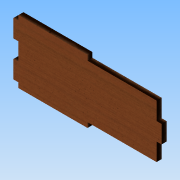
# Autodesk Inventor part: bottom2
Saved by Autodesk Inventor 2015 (Build 190159000, 159)
## iProperties
Created: 2015-12-28
Part Number: bottom2
Material: Générique
Document SubType Name: Modeling
Designer: Gregwar
Density: 1 g/cm^3
Appearance: Par défaut
Author: Gregwar
Autodesk Inventor part; units mm, degrees
ref_plane "YZ Plane" through (0, 0, 0) normal (1, 0, 0) x (0, 1, 0)
ref_plane "XZ Plane" through (0, 0, 0) normal (0, 1, 0) x (-1, 0, 0)
ref_plane "XY Plane" through (0, 0, 0) normal (0, 0, 1) x (1, 0, 0)
sketch "Esquisse1" plane through (0, 0, 0) normal (0, 1, 0) x (-1, 0, 0)
  line L0 (0, 0) -> (83, 0)
  line L1 (83, 0) -> (83, -32)
  line L2 (83, -32) -> (0, -32)
  line L3 (0, -32) -> (0, 0)
  dimension "d0" = 32
  dimension "d1" = 83
  constraints: 8 end point, 2 parallel, 1 horizontal, 1 perpendicular
  measures "d0" distance of L2.end L0.start
  measures "d1" distance of L0.start L0.end
extrude "Extrusion1" add sketch "Esquisse1" along normal blind 3
sketch "Esquisse2" plane through (0, 3, 0) normal (0, 1, 0) x (1, 0, 0)
  line L0 (-83, 0) -> (0, 0) projected
  line L1 (0, 0) -> (0, 32) projected
  line L2 (0, 32) -> (-83, 32) projected
  line L3 (-83, 32) -> (-83, 0) projected
  line L4 (-83, 0) -> (-86, 0)
  line L5 (-86, 0) -> (-86, 10.6667)
  line L6 (-86, 10.6667) -> (-83, 10.6667)
  line L7 (-83, 10.6667) -> (-83, 0)
  line L8 (-83, 16) -> (-93.4879, 16) construction
  line L9 (-83, 32) -> (0, 32)
  line L10 (-83, 0) -> (-83, 32)
  line L11 (-83, 32) -> (-86, 32)
  line L12 (-86, 32) -> (-86, 21.3333)
  line L13 (-86, 21.3333) -> (-83, 21.3333)
  line L14 (-83, 21.3333) -> (-83, 32)
  line L15 (-83, 0) -> (-41.5, 0)
  line L16 (-41.5, 0) -> (-41.5, -3)
  line L17 (-41.5, -3) -> (-83, -3)
  line L18 (-83, -3) -> (-83, 0)
  line L19 (-83, 32) -> (-41.5, 32)
  line L20 (-41.5, 32) -> (-41.5, 35)
  line L21 (-41.5, 35) -> (-83, 35)
  line L22 (-83, 35) -> (-83, 32)
  line L23 (-83, 0) -> (-86, 0)
  line L24 (-86, 0) -> (-86, -3)
  line L25 (-86, -3) -> (-83, -3)
  line L26 (-83, -3) -> (-83, 0)
  line L27 (-83, 32) -> (-86, 32)
  line L28 (-86, 32) -> (-86, 35)
  line L29 (-86, 35) -> (-83, 35)
  line L30 (-83, 35) -> (-83, 32)
  dimension "d4" = 32
  dimension "d5" = 3
  dimension "d6" = 10.6667
  dimension "d9" = 83
  dimension "d10" = 41.5
  dimension "d11" = 3
  constraints: 54 end point, 10 symmetric about line, 8 parallel, 5 horizontal, 4 perpendicular, 2 point on line, 1 midpoint
  measures "d4" distance of L2.end L0.start
  measures "d5" distance of L0.start L4.end
  measures "d6" distance of L4.end L5.end
  measures "d9" distance of L0.start L0.end
  measures "d10" distance of L16.end L17.end
  measures "d11" distance of L17.end L10.start
extrude "Extrusion2" add sketch "Esquisse2" against normal blind 3 contours L4 L5 L6 L3 | L0 L16 L17 L18 | L13 L12 L11 L3 | L22 L21 L20 L2
sketch "Esquisse6" plane through (0, 0, 0) normal (0, -1, 0) x (1, 0, 0)
  line L0 (0, 0) -> (-41.5, 0) projected
  line L1 (-41.5, 0) -> (-41.5, 3) projected
  line L2 (-41.5, 3) -> (-83, 3) projected
  line L3 (-86, 0) -> (-86, -10.6667) projected
  line L4 (-86, -10.6667) -> (-83, -10.6667) projected
  line L5 (-83, -10.6667) -> (-83, -21.3333) projected
  line L6 (-83, -21.3333) -> (-86, -21.3333) projected
  line L7 (-86, -21.3333) -> (-86, -32) projected
  line L8 (-83, -35) -> (-41.5, -35) projected
  line L9 (-41.5, -35) -> (-41.5, -32) projected
  line L10 (-41.5, -32) -> (0, -32) projected
  line L11 (0, -32) -> (0, 0) projected
  line L12 (3, -10.6667) -> (0, -10.6667)
  line L13 (0, -10.6667) -> (0, -21.3333)
  line L14 (0, -21.3333) -> (3, -21.3333)
  line L15 (3, -21.3333) -> (3, -10.6667)
  line L16 (-83, 3) -> (-83, 0) projected
  line L17 (-83, 0) -> (-86, 0) projected
  line L18 (-86, -32) -> (-83, -32) projected
  line L19 (-83, -32) -> (-83, -35) projected
  point P0 (0, -16)
  dimension "d19" = 3
  dimension "d20" = 32
  dimension "d21" = 10.6667
  constraints: 8 end point, 2 midpoint, 2 parallel, 1 horizontal, 1 perpendicular
  measures "d19" distance of L12.start L12.end
  measures "d20" distance of L10.end L0.start
  measures "d21" distance of L14.end L12.start
extrude "Extrusion5" add sketch "Esquisse6" against normal blind 3 contours L12 L15 L14 L11
equation "\"d6\" = 0.333333 * d4"
equation "\"d10\" = 0.5 * d9"
equation "\"d21\" = 0.333333 * d20"
